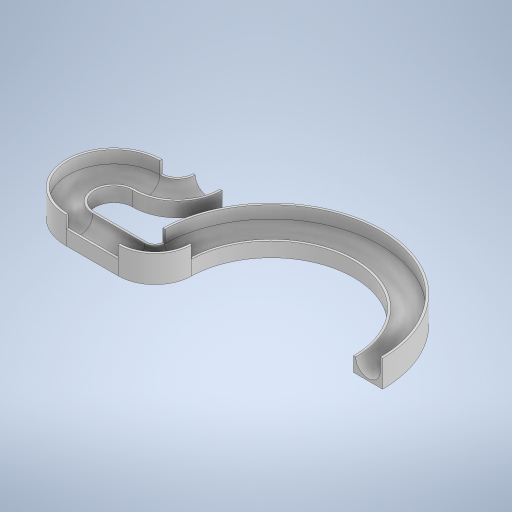
# Autodesk Inventor part: Agrupar bolinhas novamente
Saved by Autodesk Inventor 2024 (Build 280153000, 153)
## iProperties
Created: 2023-05-19
Part Number: Agrupar bolinhas novamente
Material: Genérico
Document SubType Name: Modeling
Designer: jpjoa
Density: 1 g/cm^3
Appearance: Padrão
Author: jpjoa
Autodesk Inventor part; units mm, degrees
ref_plane "YZ Plane" through (0, 0, 0) normal (1, 0, 0) x (0, 1, 0)
ref_plane "XZ Plane" through (0, 0, 0) normal (0, 1, 0) x (-1, 0, 0)
ref_plane "XY Plane" through (0, 0, 0) normal (0, 0, 1) x (1, 0, 0)
sketch "Esboço1" plane through (0, 0, 0) normal (0, 1, 0) x (-1, 0, 0)
  arc A0 (-221.4815, -24.8392) -> (-98.2625, -26.3329) centre (-159.863, -24.8392) ccw
  arc A1 (-72.9226, -1.6) -> (-98.2625, -26.3329) centre (-72.9226, -26.9474) ccw
  line L0 (-72.9226, -1.6) -> (-35, -1.6)
  arc A2 (-35, -68.4) -> (-35, -1.6) centre (-35, -35) ccw
  arc A3 (-35, -68.4) -> (-47.9358, -81.3358) centre (-35, -81.3358) ccw
  arc A4 (-35, -50.4) -> (-65.9358, -81.3358) centre (-35, -81.3358) ccw
  arc A5 (-35, -50.4) -> (-35, -19.6) centre (-35, -35) ccw
  line L1 (-35, -19.6) -> (-72.9226, -19.6)
  arc A6 (-72.9226, -19.6) -> (-80.2678, -26.7693) centre (-72.9226, -26.9474) ccw
  arc A7 (-239.4815, -24.8392) -> (-80.2678, -26.7693) centre (-159.863, -24.8392) ccw
  arc A8 (-241.0815, -24.8392) -> (-78.6683, -26.808) centre (-159.863, -24.8392) ccw
  arc A9 (-72.9226, -21.2) -> (-78.6683, -26.808) centre (-72.9226, -26.9474) ccw
  line L2 (-72.9226, -21.2) -> (-35, -21.2)
  arc A10 (-35, -48.8) -> (-35, -21.2) centre (-35, -35) ccw
  arc A11 (-35, -48.8) -> (-67.5358, -81.3358) centre (-35, -81.3358) ccw
  arc A12 (-219.8815, -24.8392) -> (-99.8621, -26.2941) centre (-159.863, -24.8392) ccw
  arc A13 (-72.9226, 0) -> (-99.8621, -26.2941) centre (-72.9226, -26.9474) ccw
  line L3 (-72.9226, 0) -> (-35, 0)
  arc A14 (-35, -70) -> (-35, 0) centre (-35, -35) ccw
  arc A15 (-35, -70) -> (-46.3358, -81.3358) centre (-35, -81.3358) ccw
  line L4 (-219.8815, -24.8392) -> (-241.0815, -24.8392)
  line L5 (-46.3358, -81.3358) -> (-67.5358, -81.3358)
  line L6 (-78.6718, -26.9474) -> (-80.2724, -26.9474)
  line L7 (-99.8815, -26.9474) -> (-98.2805, -26.9474)
  line L8 (-35, -1.6) -> (-35, 0)
  line L9 (-35, -70) -> (-35, -68.4)
  line L10 (-72.9226, -1.6) -> (-72.9226, 0)
  point P0 (0, 0)
  point P1 (-53.9613, -19.6)
  point P2 (-35, -69.2)
  point P3 (-35, -0.8)
  point P4 (-79.4721, -26.9474)
  point P5 (-99.081, -26.9474)
  point P6 (-239.4815, -24.8392)
  point P7 (-35, -68.4)
  point P8 (-35, -70)
  point P9 (0, -35)
  point P10 (-53.9613, 0)
  dimension "d10" = 18
  dimension "d11" = 30.8
  dimension "d12" = 1.6
  dimension "d13" = 1.6
  dimension "d21" = 120
  constraints: 39 point on circle, 22 end point, 16 centre point, 11 horizontal alignment, 7 vertical alignment, 6 midpoint, 5 horizontal, 3 tangent, 2 vertical, 12 other
  measures "d10" radial gap between concentric circles of A3 A4
  measures "d11" distance of L1.start A4.start
  measures "d12" radial gap between concentric circles of A7 A8
  measures "d13" radial gap between concentric circles of A1 A13
  measures "d21" horizontal distance of L4.start L7.start
extrude "Extrusão1" add sketch "Esboço1" against normal blind 1.6
extrude "Extrusão2" add sketch "Esboço1" along normal blind 18 contours L7 A12 A13 L10 A1 A0 | A7 L6 A8 L4 | L8 A14 L9 A2
extrude "Extrusão3" add sketch "Esboço1" along normal blind 9 contours L4 A12 L7 A0 | A7 A6 L1 A5 A4 L5 A11 A10 L2 A9 A8 L6 | L10 L3 L8 L0 | L9 A15 L5 A3
fillet "Arredondamento1" radius 9 8 edges at (78.0546, 0, -21.6894) (53.9613, 0, -19.6) (19.6, 0, -35) (56.8749, 0, -59.4609) (160.828, 0, -104.4519) (90.6273, 0, -8.8081) (1.6, 0, -35) (53.9613, 0, -1.6)
equation "\"d10\" = Esfera"
equation "\"d12\" = Margem"
equation "\"d13\" = Margem"
equation "\"Esfera\" = 18"
equation "\"Margem\" = 1.6"
